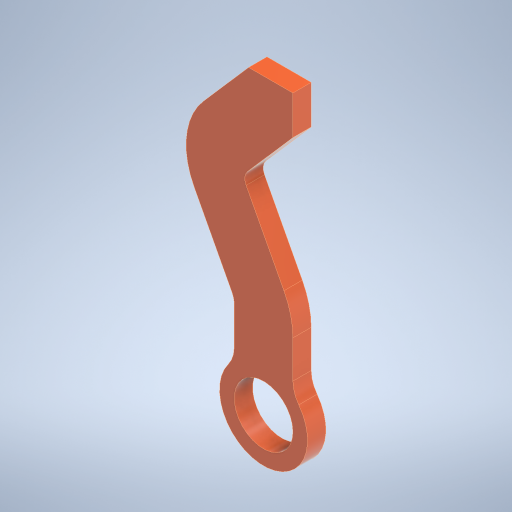
# Autodesk Inventor part: gripper
Saved by Autodesk Inventor 2023.2 (Build 272271000, 271)
## iProperties
Created: 2022-12-21
Part Number: gripper
Material: Polystyrene
Document SubType Name: Modeling
Designer: omrfrkmll
Density: 1.021 g/cm^3
Appearance: Smooth - Light Orange
Author: omrfrkmll
Autodesk Inventor part; units mm, degrees
ref_plane "YZ Plane" through (0, 0, 0) normal (1, 0, 0) x (0, 1, 0)
ref_plane "XZ Plane" through (0, 0, 0) normal (0, 1, 0) x (-1, 0, 0)
ref_plane "XY Plane" through (0, 0, 0) normal (0, 0, 1) x (1, 0, 0)
sketch "Sketch1" plane through (0, 0, 0) normal (0, 0, 1) x (1, 0, 0)
  line L0 (0, 0) -> (2.8584, 0)
  line L1 (0, 0) -> (0, 3.8884)
  circle A0 centre (0, -12.5) radius 4
  arc A1 (-4.8, -8.9) -> (4.8, -8.9) centre (0, -12.5) ccw
  line L2 (4, -1.4002) -> (4, -6.5)
  line L3 (-9.4657, 9.7101) -> (-4.3072, -0.1501)
  arc A2 (-4, -1.4002) -> (-4.3072, -0.1501) centre (-6.6968, -1.4002) ccw
  line L4 (-4, -1.4002) -> (-4, -6.5)
  line L5 (4, -6.5) -> (4, -1.4002)
  arc A3 (4, -1.4002) -> (2.7813, 3.5584) centre (-6.6968, -1.4002) ccw
  line L6 (2.7813, 3.5584) -> (-2.3771, 13.4186)
  arc A4 (-2.17, 15.1733) -> (-2.3771, 13.4186) centre (-0.9897, 14.1444) ccw
  line L7 (-2.17, 15.1733) -> (4, 22.2516)
  line L8 (4, 22.2516) -> (4, 27.5083)
  line L9 (4, 27.5083) -> (-2.0305, 27.5083)
  line L10 (-2.0305, 27.5083) -> (-8.2005, 20.4299)
  arc A5 (-8.2005, 20.4299) -> (-9.4657, 9.7101) centre (-0.9897, 14.1444) ccw
  line L11 (-4, -6.5) -> (-4, -1.4002)
  arc A6 (-4.8, -8.9) -> (-4, -6.5) centre (-8, -6.5) ccw
  arc A7 (4, -6.5) -> (4.8, -8.9) centre (8, -6.5) ccw
  dimension "d1" = 8
  dimension "d16" = 8
  dimension "d17" = 8
  dimension "d18" = 25
  dimension "d19" = 4
  dimension "d20" = 2
  dimension "d21" = 2.8003
  dimension "d22" = 13.3936
  dimension "d23" = 1.9794
  dimension "d24" = 28.2888
  dimension "d25" = 0
  constraints: 24 end point, 14 point on circle, 12 tangent, 8 centre point, 6 parallel, 3 vertical, 2 coincident, 1 equal radius, 1 horizontal, 1 perpendicular
  measures "d1" diameter of A0
  measures "d16" diameter of L2 L1
  measures "d17" diameter of L4 L1
  measures "d18" diameter of A0.centre L0
  measures "d19" radius of A6
  measures "d20" radial gap between concentric circles of A1 A0
  measures "d21" diameter of A2.centre L0
  measures "d22" diameter of A2.centre L1
  measures "d23" diameter of A5.centre L1
  measures "d24" diameter of A5.centre L0
  measures "d25" distance between parallel lines of L5 L8
extrude "Extrusion1" add sketch "Sketch1" along normal blind 2.5
body "Solid1"
